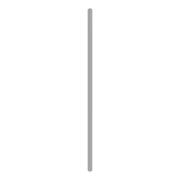
# Autodesk Inventor part: MSI-102
Saved by Autodesk Inventor 2020.3 (Build 243373000, 373)
## iProperties
Created: 2021-02-10
Part Number: MSI-102
Material: Aço inoxidável AISI 304
Document SubType Name: Modeling
Designer: Adriano
Density: 8 g/cm^3
Appearance: Cromado - Acetinado
Author: Adriano
Autodesk Inventor part; units mm, degrees
ref_plane "YZ Plane" through (0, 0, 0) normal (1, 0, 0) x (0, 1, 0)
ref_plane "XZ Plane" through (0, 0, 0) normal (0, 1, 0) x (-1, 0, 0)
ref_plane "XY Plane" through (0, 0, 0) normal (0, 0, 1) x (1, 0, 0)
sketch "Esboço1" plane through (0, 0, 0) normal (0, 1, 0) x (-1, 0, 0)
  line L0 (-18.5, 20) -> (18.5, 20)
  line L1 (20, 18.5) -> (20, -18.5)
  line L2 (18.5, -20) -> (-18.5, -20)
  line L3 (-20, -18.5) -> (-20, 18.5)
  line L4 (-20, 20) -> (20, -20) construction
  line L5 (20, 20) -> (-20, -20) construction
  line L6 (-18.5, -18.5) -> (18.5, -18.5)
  line L7 (18.5, -18.5) -> (18.5, 18.5)
  line L8 (18.5, 18.5) -> (-18.5, 18.5)
  line L9 (-18.5, 18.5) -> (-18.5, -18.5)
  line L10 (-18.5, -18.5) -> (18.5, 18.5) construction
  line L11 (18.5, -18.5) -> (-18.5, 18.5) construction
  arc A0 (20, 18.5) -> (18.5, 20) centre (18.5, 18.5) ccw
  arc A1 (-18.5, 20) -> (-20, 18.5) centre (-18.5, 18.5) ccw
  arc A2 (-20, -18.5) -> (-18.5, -20) centre (-18.5, -18.5) ccw
  arc A3 (18.5, -20) -> (20, -18.5) centre (18.5, -18.5) ccw
  point P0 (0, 0)
  dimension "d0" = 40
  dimension "d1" = 40
  dimension "d2" = 1.5
  dimension "d3" = 1.5
  constraints: 24 end point, 9 point on line, 8 point on circle, 8 tangent, 4 centre point, 4 midpoint, 4 parallel, 3 equal radius, 2 horizontal, 2 perpendicular
  measures "d0" distance of L4.end L5.end
  measures "d1" distance of L5.start L4.end
  measures "d2" distance between parallel lines of L1 L7
  measures "d3" radius of A0
extrude "Extrusão1" add sketch "Esboço1" along normal mid plane 2500
equation "\"d3\" = d2"
